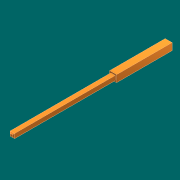
# Autodesk Inventor part: pin
Saved by Autodesk Inventor 2016 SP1 (Build 200210100, 210)
## iProperties
Created: 2016-04-06
Part Number: pin
Material: Gold
Document SubType Name: Modeling
Designer: sawai
Density: 19.3 g/cm^3
Appearance: Metal 1600F Hot
Author: sawai
Autodesk Inventor part; units mm, degrees
ref_plane "YZ Plane" through (0, 0, 0) normal (1, 0, 0) x (0, 1, 0)
ref_plane "XZ Plane" through (0, 0, 0) normal (0, 1, 0) x (-1, 0, 0)
ref_plane "XY Plane" through (0, 0, 0) normal (0, 0, 1) x (1, 0, 0)
sketch "Sketch1" plane through (0, 0, 0) normal (0, 1, 0) x (-1, 0, 0)
  line L0 (-0.5, 0.5) -> (0.5, 0.5)
  line L1 (0.5, 0.5) -> (0.5, -0.5)
  line L2 (0.5, -0.5) -> (-0.5, -0.5)
  line L3 (-0.5, -0.5) -> (-0.5, 0.5)
  line L4 (-0.5, 0.5) -> (0.5, -0.5) construction
  line L5 (0.5, 0.5) -> (-0.5, -0.5) construction
  point P0 (0, 0)
  dimension "d0" = 1
  dimension "d1" = 1
  constraints: 12 end point, 2 midpoint, 2 parallel, 1 horizontal, 1 perpendicular
  measures "d0" distance of L1.end L2.end
  measures "d1" distance of L0.end L1.end
extrude "Extrusion1" add sketch "Sketch1" along normal blind 8
sketch "Sketch2" plane through (0, 0, 0) normal (0, -1, 0) x (1, 0, 0)
  line L0 (-0.32, 0.32) -> (0.32, 0.32)
  line L1 (0.32, 0.32) -> (0.32, -0.32)
  line L2 (0.32, -0.32) -> (-0.32, -0.32)
  line L3 (-0.32, -0.32) -> (-0.32, 0.32)
  line L4 (-0.32, 0.32) -> (0.32, -0.32) construction
  line L5 (0.32, 0.32) -> (-0.32, -0.32) construction
  point P0 (0, 0)
  dimension "d4" = 0.64
  dimension "d5" = 0.64
  constraints: 12 end point, 2 midpoint, 2 parallel, 1 horizontal, 1 perpendicular
  measures "d4" distance of L1.end L2.end
  measures "d5" distance of L0.end L1.end
extrude "Extrusion2" add sketch "Sketch2" along normal blind 14.65
chamfer "Chamfer1" distance 0.155 angle 45 4 edges at (0, -14.65, 0.32) (0.32, -14.65, 0) (0, -14.65, -0.32) (-0.32, -14.65, 0)
sketch "Sketch3" plane through (0, 8, 0) normal (0, 1, 0) x (1, 0, 0)
  line L0 (0.32, 0.32) -> (-0.32, 0.32)
  line L1 (-0.32, 0.32) -> (-0.32, -0.32)
  line L2 (-0.32, -0.32) -> (0.32, -0.32)
  line L3 (0.32, -0.32) -> (0.32, 0.32)
  line L4 (0.32, 0.32) -> (-0.32, -0.32) construction
  line L5 (-0.32, 0.32) -> (0.32, -0.32) construction
  point P0 (0, 0)
  dimension "d11" = 0.64
  dimension "d12" = 0.64
  constraints: 12 end point, 2 midpoint, 2 parallel, 1 horizontal, 1 perpendicular
  measures "d11" distance of L2.end L1.end
  measures "d12" distance of L1.end L0.end
extrude "Extrusion3" cut sketch "Sketch3" against normal blind 6
body "Solid1"
